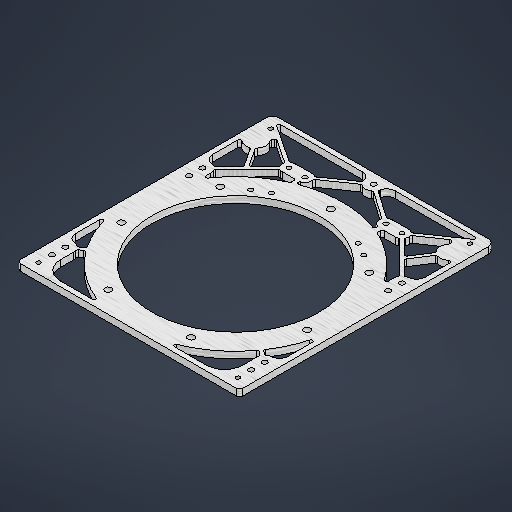
# Autodesk Inventor part: PLATE,SHOOTER,BOTTOM
Saved by Autodesk Inventor 2026.1 (Build 301233020, 233B)
## iProperties
Created: 2026-01-27
Part Number: PLATE,SHOOTER,BOTTOM
Material: Aluminum 7075
Document SubType Name: Sheet Metal
Designer: Owen L
Density: 2.81 g/cm^3
Appearance: Satin - Brushed Heavy
Mass: 376.468 g
Surface Area: 643.616 cm^2
Volume: 133.974 cm^3
Sheet Metal Rule: Default
Author: Owen L
Autodesk Inventor part; units mm, degrees
ref_plane "YZ Plane" through (0, 0, 0) normal (1, 0, 0) x (0, 1, 0)
ref_plane "XZ Plane" through (0, 0, 0) normal (0, 1, 0) x (-1, 0, 0)
ref_plane "XY Plane" through (0, 0, 0) normal (0, 0, 1) x (1, 0, 0)
sketch "Sketch1" plane through (0, 0, 0) normal (0, 1, 0) x (-1, 0, 0)
  line L0 (-105.7173, 139.7) -> (105.7173, 139.7)
  line L1 (105.7173, 139.7) -> (105.7173, -139.7)
  line L2 (105.7173, -139.7) -> (-105.7173, -139.7)
  line L3 (-105.7173, -139.7) -> (-105.7173, 139.7)
  line L4 (-105.7173, 139.7) -> (105.7173, -139.7) construction
  line L5 (105.7173, 139.7) -> (-105.7173, -139.7) construction
  circle A0 centre (0, 37.7949) radius 79.375
  point P0 (0, 0)
  dimension "d0" = 211.4347
  dimension "d1" = 279.4
  dimension "d2" = 158.75
  dimension "d3" = 101.9051
  measures "d0" distance of L1.end L2.end
  measures "d1" distance of L0.end L1.end
  measures "d2" diameter of A0
  measures "d3" distance from line of L0 A0.centre
extrude "Plate1" add sketch "Sketch1" along normal blind 6.35
sketch "Sketch2" plane through (0, 0, 0) normal (0, -1, 0) x (1, 0, 0)
  point P0 (0, 0)
  point P1 (-41.275, -37.3842)
  point P2 (-38.4175, -66.5942)
  point P3 (-53.6575, -66.5942)
  point P4 (-53.6575, -30.3992)
  dimension "d7" = 37.3842
  dimension "d11" = 41.275
  dimension "d12" = 6.985
  dimension "d13" = 29.21
  dimension "d14" = 2.8575
  dimension "d15" = 12.3825
  constraints: 1 horizontal alignment, 1 vertical alignment
  measures "d7" vertical distance of point (-41.275, -37.384) point (0, 0)
  measures "d11" horizontal distance of point (0, 0) point (-41.275, -37.384)
  measures "d12" vertical distance of point (-53.658, -30.399) point (-41.275, -37.384)
  measures "d13" vertical distance of point (-38.418, -66.594) point (-41.275, -37.384)
  measures "d14" horizontal distance of point (-38.418, -66.594) point (-41.275, -37.384)
  measures "d15" horizontal distance of point (-53.658, -66.594) point (-41.275, -37.384)
hole "Hole1" at (-41.275, 0, -37.3842) at (-38.4175, 0, -66.5942) at (-53.6575, 0, -66.5942) at (-53.6575, 0, -30.3992) direction (0, 1, 0) diameter 4.2926 depth 6.35 clearance for "Flat Head Machine Screw" size "M4" standard "Ansi Metric M Profile"
mirror "Mirror1" about plane through (0, 0, 0) normal (1, 0, 0) of "Hole1"
sketch "Sketch3" plane through (0, 6.35, 0) normal (0, 1, 0) x (1, 0, 0)
  line L0 (105.7173, -139.7) -> (-105.7173, -139.7) construction
  line L1 (105.7173, 139.7) -> (105.7173, -139.7) construction
  line L2 (-105.7173, 139.7) -> (105.7173, 139.7) construction
  line L3 (0, -139.7) -> (0, 139.7) construction
  point P0 (0, 0)
  point P1 (94.6048, -117.475)
  point P2 (94.6048, -104.775)
  point P3 (94.6048, 12.7)
  point P4 (94.6048, 25.4)
  point P5 (-87.3125, 139.7)
  point P6 (-94.6048, -117.475)
  point P7 (-94.6048, -104.775)
  point P8 (-94.6048, 12.7)
  point P9 (-94.6048, 25.4)
  dimension "d23" = 22.225
  dimension "d24" = 12.7
  dimension "d25" = 11.1125
  dimension "d26" = 12.7
  dimension "d60" = 152.4
  constraints: 4 symmetric about line, 3 vertical alignment, 2 end point, 2 midpoint
  measures "d23" distance from line of L0 point (94.605, -117.475)
  measures "d24" distance of point (94.605, -104.775) point (94.605, -117.475)
  measures "d25" distance from line of L1 point (94.605, -117.475)
  measures "d26" distance of point (94.605, 25.4) point (94.605, 12.7)
  measures "d60" distance from line of L0 point (94.605, 12.7)
hole "Hole2" at (94.6048, 6.35, 117.475) at (94.6048, 6.35, 104.775) at (94.6048, 6.35, -12.7) at (94.6048, 6.35, -25.4) at (-94.6048, 6.35, -25.4) at (-94.6048, 6.35, -12.7) at (-94.6048, 6.35, 104.775) at (-94.6048, 6.35, 117.475) direction (0, -1, 0) diameter 4.9784 depth 6.35 clearance for "Flat Head Machine Screw (82)" size "#10" standard "Ansi Unified Screw Threads"
sketch "Sketch5" plane through (0, 6.35, 0) normal (0, 1, 0) x (1, 0, 0)
  line L0 (-105.7173, 139.7) -> (-105.7173, -139.7) projected
  line L1 (105.7173, 139.7) -> (105.7173, -139.7) projected
  line L2 (-105.7173, 139.7) -> (105.7173, 139.7)
  line L3 (105.7173, 139.7) -> (105.7173, 102.9208)
  line L4 (105.7173, 102.9208) -> (-105.7173, 102.9208)
  line L5 (-105.7173, 102.9208) -> (-105.7173, 139.7)
  point P0 (0, 0)
  dimension "d61" = 36.7792
  constraints: 8 end point, 2 parallel, 1 horizontal, 1 perpendicular, 1 point on line
  measures "d61" distance of L2.end L3.end
extrude "Cut2" cut sketch "Sketch5" against normal blind 6.35
fillet "Corner Round3" radius 6.35 2 edges at (-105.7173, 3.175, -102.9208) (105.7173, 3.175, -102.9208)
fillet "Corner Round3" radius 3.175 2 edges at (-105.7173, 3.175, 139.7) (105.7173, 3.175, 139.7)
sketch "Sketch6" plane through (0, 6.35, 0) normal (0, 1, 0) x (1, 0, 0)
  line L0 (99.3673, 102.9208) -> (-99.3673, 102.9208) projected
  point P0 (0, 0)
  point P1 (0, 93.3958)
  dimension "d66" = 9.525
  constraints: 1 vertical alignment
  measures "d66" distance from line of L0 point (0, 93.396)
hole "Hole3" at (0, 6.35, -93.3958) direction (0, -1, 0) diameter 4.9784 end through all clearance for "Flat Head Machine Screw (82)" size "#10" standard "Ansi Unified Screw Threads"
sketch "Sketch7" plane through (0, 6.35, 0) normal (0, 1, 0) x (1, 0, 0)
  circle A0 centre (0, 93.3958) radius 2.4892 projected
  arc A1 (102.5423, -139.7) -> (105.7173, -136.525) centre (102.5423, -136.525) ccw projected
  line L0 (105.7173, 96.5708) -> (105.7173, -136.525) projected
  arc A2 (105.7173, 96.5708) -> (99.3673, 102.9208) centre (99.3673, 96.5708) ccw projected
  line L1 (99.3673, 102.9208) -> (-99.3673, 102.9208) projected
  arc A3 (-99.3673, 102.9208) -> (-105.7173, 96.5708) centre (-99.3673, 96.5708) ccw projected
  line L2 (-105.7173, -136.525) -> (-105.7173, 96.5708) projected
  arc A4 (-105.7173, -136.525) -> (-102.5423, -139.7) centre (-102.5423, -136.525) ccw projected
  line L3 (102.5423, -139.7) -> (-102.5423, -139.7) projected
  circle A5 centre (-94.6048, -117.475) radius 2.4892 projected
  circle A6 centre (-94.6048, -104.775) radius 2.4892 projected
  circle A7 centre (-94.6048, 12.7) radius 2.4892 projected
  circle A8 centre (-94.6048, 25.4) radius 2.4892 projected
  circle A9 centre (94.6048, 25.4) radius 2.4892 projected
  circle A10 centre (94.6048, 12.7) radius 2.4892 projected
  circle A11 centre (94.6048, -104.775) radius 2.4892 projected
  circle A12 centre (94.6048, -117.475) radius 2.4892 projected
  circle A13 centre (53.6575, 30.3992) radius 2.1463 projected
  circle A14 centre (53.6575, 66.5942) radius 2.1463 projected
  circle A15 centre (38.4175, 66.5942) radius 2.1463 projected
  circle A16 centre (41.275, 37.3842) radius 2.1463 projected
  circle A17 centre (-53.6575, 30.3992) radius 2.1463 projected
  circle A18 centre (-53.6575, 66.5942) radius 2.1463 projected
  circle A19 centre (-38.4175, 66.5942) radius 2.1463 projected
  circle A20 centre (-41.275, 37.3842) radius 2.1463 projected
  circle A21 centre (0, -37.7949) radius 79.375 projected
  arc A22 (-99.3673, 98.1583) -> (-100.9548, 96.5708) centre (-99.3673, 96.5708) ccw
  line L4 (-99.3673, 98.1583) -> (99.3673, 98.1583)
  arc A23 (100.9548, 96.5708) -> (99.3673, 98.1583) centre (99.3673, 96.5708) ccw
  line L5 (100.9548, 96.5708) -> (100.9548, -134.9375)
  line L6 (100.9548, -134.9375) -> (-100.9548, -134.9375)
  line L7 (-100.9548, -134.9375) -> (-100.9548, 96.5708)
  circle A24 centre (0, -37.7949) radius 101.6
  circle A25 centre (94.6048, 12.7) radius 7.9375
  circle A26 centre (94.6048, 25.4) radius 7.9375
  circle A27 centre (-94.6048, 12.7) radius 7.9375
  circle A28 centre (-94.6048, 25.4) radius 7.9375
  circle A29 centre (-94.6048, -117.475) radius 7.9375
  circle A30 centre (-94.6048, -104.775) radius 7.9375
  circle A31 centre (94.6048, -117.475) radius 7.9375
  circle A32 centre (94.6048, -104.775) radius 7.9375
  circle A33 centre (53.6575, 66.5942) radius 6.35
  circle A34 centre (38.4175, 66.5942) radius 6.35
  circle A35 centre (0, 93.3958) radius 7.9375
  circle A36 centre (-38.4175, 66.5942) radius 6.35
  circle A37 centre (-53.6575, 66.5942) radius 2.1463 projected
  circle A38 centre (-53.6575, 66.5942) radius 6.35
  line L8 (86.6673, -117.475) -> (86.6673, -104.775)
  line L9 (-86.6673, -117.475) -> (-86.6673, -104.775)
  line L10 (86.6673, 25.4) -> (86.6673, 12.7)
  line L11 (53.6575, 60.2442) -> (38.4175, 60.2442)
  line L12 (38.4175, 72.9442) -> (53.6575, 72.9442)
  line L13 (-38.4175, 72.9442) -> (-53.6575, 72.9442)
  line L14 (-53.6575, 60.2442) -> (-38.4175, 60.2442)
  line L15 (-86.6673, 12.7) -> (-86.6673, 25.4)
  arc A39 (-86.6673, -117.475) -> (-69.2048, -134.9375) centre (-69.2048, -117.475) ccw
  arc A40 (69.2048, -134.9375) -> (86.6673, -117.475) centre (69.2048, -117.475) ccw
  arc A41 (93.8111, 33.2977) -> (86.6673, 25.4) centre (94.6048, 25.4) ccw
  arc A42 (93.8111, 33.2977) -> (100.9548, 41.1954) centre (93.0173, 41.1954) ccw
  arc A43 (-86.6673, 25.4) -> (-93.8111, 33.2977) centre (-94.6048, 25.4) ccw
  arc A44 (-100.9548, 41.1954) -> (-93.8111, 33.2977) centre (-93.0173, 41.1954) ccw
  line L16 (0, 85.4583) -> (-7.6538, 85.4583) construction
  line L17 (0, 85.4583) -> (6.7881, 85.4583) construction
  arc A45 (-7.7771, 91.8083) -> (0, 85.4583) centre (0, 93.3958) ccw
  arc A46 (-7.7771, 91.8083) -> (-15.5543, 98.1583) centre (-15.5543, 90.2208) ccw
  arc A47 (0, 85.4583) -> (7.7771, 91.8083) centre (0, 93.3958) ccw
  arc A48 (15.5543, 98.1583) -> (7.7771, 91.8083) centre (15.5543, 90.2208) ccw
  arc A49 (-86.6673, -104.775) -> (-93.8111, -96.8773) centre (-94.6048, -104.775) ccw
  arc A50 (-100.9548, -88.9796) -> (-93.8111, -96.8773) centre (-93.0173, -88.9796) ccw
  arc A51 (93.8111, -96.8773) -> (86.6673, -104.775) centre (94.6048, -104.775) ccw
  arc A52 (93.8111, -96.8773) -> (100.9548, -88.9796) centre (93.0173, -88.9796) ccw
  arc A53 (1.4242, 91.3543) -> (-1.4242, 95.4373) centre (0, 93.3958) ccw
  line L18 (-53.6575, 66.5942) -> (-94.6048, 25.4) construction
  line L19 (-54.7834, 67.7134) -> (-95.7307, 26.5192)
  line L20 (-93.4789, 24.2808) -> (-52.5316, 65.475)
  arc A54 (-52.5316, 65.475) -> (-54.7834, 67.7134) centre (-53.6575, 66.5942) ccw
  arc A55 (-95.7307, 26.5192) -> (-93.4789, 24.2808) centre (-94.6048, 25.4) ccw
  line L21 (-53.6575, 66.5942) -> (-104.477, 100.341) construction
  line L22 (-52.7793, 67.9167) -> (-103.5988, 101.6634)
  line L23 (-105.3552, 99.0185) -> (-54.5357, 65.2717)
  arc A56 (-54.5357, 65.2717) -> (-52.7793, 67.9167) centre (-53.6575, 66.5942) ccw
  arc A57 (-103.5988, 101.6634) -> (-105.3552, 99.0185) centre (-104.477, 100.341) ccw
  line L24 (-38.4175, 66.5942) -> (-41.275, 37.3842) construction
  line L25 (-39.9975, 66.7488) -> (-42.855, 37.5388)
  line L26 (-39.695, 37.2296) -> (-36.8375, 66.4396)
  arc A58 (-36.8375, 66.4396) -> (-39.9975, 66.7488) centre (-38.4175, 66.5942) ccw
  arc A59 (-42.855, 37.5388) -> (-39.695, 37.2296) centre (-41.275, 37.3842) ccw
  line L27 (38.4175, 66.5942) -> (41.275, 37.3842) construction
  line L28 (36.2814, 66.3852) -> (39.1389, 37.1752)
  line L29 (43.4111, 37.5932) -> (40.5536, 66.8032)
  arc A60 (40.5536, 66.8032) -> (36.2814, 66.3852) centre (38.4175, 66.5942) ccw
  arc A61 (39.1389, 37.1752) -> (43.4111, 37.5932) centre (41.275, 37.3842) ccw
  line L30 (38.4175, 66.5942) -> (0, 93.3958) construction
  line L31 (39.3258, 67.8962) -> (0.9083, 94.6978)
  line L32 (-0.9083, 92.0938) -> (37.5092, 65.2922)
  arc A62 (37.5092, 65.2922) -> (39.3258, 67.8962) centre (38.4175, 66.5942) ccw
  arc A63 (0.9083, 94.6978) -> (-0.9083, 92.0938) centre (0, 93.3958) ccw
  line L33 (53.6575, 66.5942) -> (94.6048, 25.4) construction
  line L34 (52.5316, 65.475) -> (93.4789, 24.2808)
  line L35 (95.7307, 26.5192) -> (54.7834, 67.7134)
  arc A64 (54.7834, 67.7134) -> (52.5316, 65.475) centre (53.6575, 66.5942) ccw
  arc A65 (93.4789, 24.2808) -> (95.7307, 26.5192) centre (94.6048, 25.4) ccw
  line L36 (53.6575, 66.5942) -> (103.8575, 101.0609) construction
  line L37 (54.5561, 65.2855) -> (104.756, 99.7522)
  line L38 (102.9589, 102.3697) -> (52.7589, 67.9029)
  arc A66 (52.7589, 67.9029) -> (54.5561, 65.2855) centre (53.6575, 66.5942) ccw
  arc A67 (104.756, 99.7522) -> (102.9589, 102.3697) centre (103.8575, 101.0609) ccw
  line L39 (-38.4175, 66.5942) -> (0, 93.3958) construction
  line L40 (-37.5092, 65.2922) -> (0.9083, 92.0938)
  line L41 (-0.9083, 94.6978) -> (-39.3258, 67.8962)
  arc A68 (-39.3258, 67.8962) -> (-37.5092, 65.2922) centre (-38.4175, 66.5942) ccw
  arc A69 (0.9083, 92.0938) -> (-0.9083, 94.6978) centre (0, 93.3958) ccw
  line L42 (-94.6048, -104.775) -> (0, -37.7949) construction
  line L43 (-93.6875, -106.0706) -> (0.9173, -39.0906)
  line L44 (-0.9173, -36.4993) -> (-95.5222, -103.4794)
  arc A70 (-95.5222, -103.4794) -> (-93.6875, -106.0706) centre (-94.6048, -104.775) ccw
  arc A71 (0.9173, -39.0906) -> (-0.9173, -36.4993) centre (0, -37.7949) ccw
  line L45 (94.6048, -104.775) -> (0, -37.7949) construction
  line L46 (95.5222, -103.4794) -> (0.9173, -36.4993)
  line L47 (-0.9173, -39.0906) -> (93.6875, -106.0706)
  arc A72 (93.6875, -106.0706) -> (95.5222, -103.4794) centre (94.6048, -104.775) ccw
  arc A73 (0.9173, -36.4993) -> (-0.9173, -39.0906) centre (0, -37.7949) ccw
  circle A74 centre (-92.2553, 73.7108) radius 9.525
  line L48 (-92.2553, 73.7108) -> (-83.7232, 86.5594) construction
  line L49 (-90.9329, 72.8326) -> (-82.4007, 85.6812)
  line L50 (-85.0457, 87.4376) -> (-93.5778, 74.589)
  arc A75 (-93.5778, 74.589) -> (-90.9329, 72.8326) centre (-92.2553, 73.7108) ccw
  arc A76 (-82.4007, 85.6812) -> (-85.0457, 87.4376) centre (-83.7232, 86.5594) ccw
  line L51 (-92.2553, 73.7108) -> (-74.1312, 45.9971) construction
  line L52 (-93.5839, 72.8419) -> (-75.4598, 45.1282)
  line L53 (-72.8026, 46.866) -> (-90.9267, 74.5797)
  arc A77 (-90.9267, 74.5797) -> (-93.5839, 72.8419) centre (-92.2553, 73.7108) ccw
  arc A78 (-75.4598, 45.1282) -> (-72.8026, 46.866) centre (-74.1312, 45.9971) ccw
  line L54 (0, 102.9208) -> (0, -139.7) construction
  circle A79 centre (92.2553, 73.7108) radius 9.525
  line L55 (90.9329, 72.8326) -> (82.4007, 85.6812)
  line L56 (85.0457, 87.4376) -> (93.5778, 74.589)
  line L57 (92.2553, 73.7108) -> (74.1312, 45.9971) construction
  line L58 (93.5839, 72.8419) -> (75.4598, 45.1282)
  line L59 (72.8026, 46.866) -> (90.9267, 74.5797)
  point P0 (0, 0)
  point P1 (-74.1312, 45.9971)
  point P2 (-79.0672, 83.4676)
  point P3 (-100.4899, 97.6933)
  point P4 (-39.8463, 51.9892)
  point P5 (39.8463, 51.9892)
  point P6 (19.2088, 79.995)
  point P7 (74.1312, 45.9971)
  point P8 (78.7575, 83.8276)
  point P9 (-19.2088, 79.995)
  point P10 (-47.3024, -71.285)
  point P11 (47.3024, -71.285)
  point P12 (83.8284, -95.2002)
  point P13 (89.1748, -98.9855)
  point P14 (100.9548, -49.2265)
  point P15 (87.3402, -101.5767)
  point P16 (81.9938, -97.7915)
  point P17 (29.7638, -134.9375)
  point P18 (100.8696, 97.0839)
  point P19 (59.6247, 68.7656)
  point P20 (59.1179, 63.3528)
  point P21 (90.248, 32.0349)
  point P22 (93.8111, 33.2977)
  point P23 (87.9962, 29.7966)
  point P24 (56.8661, 61.1145)
  point P25 (41.1952, 60.2442)
  point P26 (41.7237, 54.8425)
  point P27 (86.6673, 15.2271)
  point P28 (57.8276, 71.383)
  point P29 (96.8252, 98.1583)
  point P30 (7.7771, 91.8083)
  point P31 (7.2866, 90.248)
  point P32 (34.2833, 71.414)
  point P33 (-5.47, 87.644)
  point P34 (-32.4667, 68.8101)
  point P35 (-37.4362, 60.3205)
  point P36 (-37.8091, 56.5079)
  point P37 (37.2249, 56.74)
  point P38 (36.8633, 60.4374)
  point P39 (32.4667, 68.8101)
  point P40 (5.47, 87.644)
  point P41 (-34.2833, 71.414)
  point P42 (-7.2866, 90.248)
  point P43 (-7.7771, 91.8083)
  point P44 (-98.3204, 98.1583)
  point P45 (-57.9012, 71.3179)
  point P46 (-59.6576, 68.6729)
  point P47 (-100.9548, 96.0965)
  point P48 (-93.8111, 33.2977)
  point P49 (-90.248, 32.0349)
  point P50 (-59.1179, 63.3528)
  point P51 (-41.1366, 55.1047)
  point P52 (-40.6338, 60.2442)
  point P53 (-56.8661, 61.1145)
  point P54 (-87.9962, 29.7966)
  point P55 (-86.6673, 15.2271)
  point P56 (-89.1748, -98.9855)
  point P57 (-83.8284, -95.2002)
  point P58 (-100.9548, -49.2265)
  point P59 (-29.7638, -134.9375)
  point P60 (-81.9938, -97.7915)
  point P61 (-87.3402, -101.5767)
  point P62 (-87.9893, 80.1351)
  point P63 (-83.1933, 59.854)
  point P64 (-76.1635, 46.2043)
  point P65 (-88.4436, 64.9818)
  point P66 (-100.9548, 69.8321)
  point P67 (-88.3824, 82.4129)
  point P68 (-85.9239, 86.1151)
  point P69 (-85.7864, 66.7195)
  point P70 (-73.8753, 48.5063)
  point P71 (-83.2789, 84.3587)
  point P72 (-85.7374, 80.6565)
  point P73 (85.7864, 66.7195)
  point P74 (85.7374, 80.6565)
  point P75 (82.9836, 84.8035)
  point P76 (73.8753, 48.5063)
  point P77 (100.9548, 69.8321)
  point P78 (88.4436, 64.9818)
  point P79 (76.1635, 46.2043)
  point P80 (85.6013, 86.6008)
  point P81 (88.3824, 82.4129)
  point P82 (-82.845, 87.8819)
  point P83 (-100.9548, 77.5895)
  point P84 (100.9548, 77.5895)
  dimension "d75" = 15.875
  dimension "d74" = 4.7625
  dimension "d76" = 12.7
  dimension "d77" = 7.9375
  dimension "d78" = 4.9784
  dimension "d79" = 3.175
  dimension "d80" = 3.175
  dimension "d81" = 3.175
  dimension "d82" = 4.2926
  dimension "d83" = 3.175
  dimension "d84" = 3.175
  dimension "d85" = 3.175
  dimension "d86" = 3.175
  dimension "d87" = 3.175
  dimension "d88" = 3.175
  dimension "d92" = 13.462
  dimension "d93" = 29.21
  dimension "d94" = 3.175
  dimension "d95" = 3.175
  dimension "d96" = 19.05
  dimension "d97" = 19.05
  dimension "d103" = 203.2
  constraints: 138 end point, 93 point on circle, 67 tangent, 48 centre point, 23 equal radius, 16 point on line, 15 midpoint, 14 coincident, 12 parallel, 10 symmetric about line, 5 vertical, 4 horizontal, 4 horizontal alignment, 1 perpendicular, 28 other
  measures "d74" distance between parallel lines of L2 L7
  measures "d76" diameter of A33
  measures "d77" radius of A42
  measures "d78" diameter of A53
  measures "d79" diameter of A55
  measures "d80" diameter of A57
  measures "d81" diameter of A59
  measures "d82" diameter of A61
  measures "d83" diameter of A63
  measures "d84" diameter of A65
  measures "d85" diameter of A67
  measures "d86" diameter of A69
  measures "d87" diameter of A71
  measures "d88" diameter of A73
  measures "d92" distance from line of L2 L48.start
  measures "d93" distance from line of L1 L48.start
  measures "d94" diameter of A76
  measures "d95" diameter of A78
  measures "d96" diameter of A74
  measures "d97" diameter of A79
  measures "d103" diameter of A24
extrude "Cut3" cut sketch "Sketch7" against normal blind 6.35 contours L32 A34 L28 A24 L26 A36 L40 A35 | A35 A48 L4 L38 A33 L12 A34 L31 | L41 A36 L13 A38 L22 L4 A46 A35 | L11 A33 L34 A26 L10 A24 L29 | A24 L15 A28 L20 A38 L14 L25 | L37 L55 A79 L59 L35 A33 | A38 L19 L53 A74 L49 L23 | L35 L58 A79 L5 A42 A26 | L5 A52 A32 L46 A24 | A28 A44 L7 A74 L52 L19 | A24 L44 A30 A50 L7 | L47 A32 L8 A40 L6 A24 | A24 L6 A39 L9 A30 L43
fillet "Corner Round4" radius 1.5875 58 edges at (-100.9548, 3.175, 49.2265) (-89.1748, 3.175, 98.9855) (-83.8284, 3.175, 95.2002) (-81.9938, 3.175, 97.7915) (-87.3402, 3.175, 101.5767) (-29.7638, 3.175, 134.9375) (87.3402, 3.175, 101.5767) (89.1748, 3.175, 98.9855) (81.9938, 3.175, 97.7915) (29.7638, 3.175, 134.9375) (83.8284, 3.175, 95.2002) (100.9548, 3.175, 49.2265) (87.9962, 3.175, -29.7966) (90.248, 3.175, -32.0349) (56.8661, 3.175, -61.1145) (59.1179, 3.175, -63.3528) (32.4667, 3.175, -68.8101) (36.8633, 3.175, -60.4374) (37.2249, 3.175, -56.74) (41.7237, 3.175, -54.8425) (-87.9962, 3.175, -29.7966) (-32.4667, 3.175, -68.8101) (-5.47, 3.175, -87.644) (5.47, 3.175, -87.644) (-41.1366, 3.175, -55.1047) (-86.6673, 3.175, -15.2271) (7.2866, 3.175, -90.248) (34.2833, 3.175, -71.414) (41.1952, 3.175, -60.2442) (57.8276, 3.175, -71.383) (-98.3204, 3.175, -98.1583) (-34.2833, 3.175, -71.414) (-7.2866, 3.175, -90.248) (59.6247, 3.175, -68.7656) (96.8252, 3.175, -98.1583) (86.6673, 3.175, -15.2271) (-59.6576, 3.175, -68.6729) (-57.9012, 3.175, -71.3179) (-37.4362, 3.175, -60.3205) (-37.8091, 3.175, -56.5079) (-40.6338, 3.175, -60.2442) (-59.1179, 3.175, -63.3528) (-90.248, 3.175, -32.0349) (-56.8661, 3.175, -61.1145) (-100.9548, 3.175, -69.8321) (-88.4436, 3.175, -64.9818) (-76.1635, 3.175, -46.2043) (-85.7864, 3.175, -66.7195) (-85.7374, 3.175, -80.6565) (-83.2789, 3.175, -84.3587) (-73.8753, 3.175, -48.5063) (85.7374, 3.175, -80.6565) (85.7864, 3.175, -66.7195) (73.8753, 3.175, -48.5063) (82.9836, 3.175, -84.8035) (76.1635, 3.175, -46.2043) (88.4436, 3.175, -64.9818) (100.9548, 3.175, -69.8321)
sketch "Sketch8" plane through (0, 0, 0) normal (0, -1, 0) x (1, 0, 0)
  circle A0 centre (0, 37.7949) radius 79.375 projected
  point P0 (0, 0)
  point P1 (0, -52.6926)
  point P2 (70.746, -18.6231)
  point P3 (88.2188, 57.9303)
  point P4 (39.2611, 119.3214)
  point P5 (-39.2611, 119.3214)
  point P6 (-88.2188, 57.9303)
  point P7 (-70.746, -18.6231)
  dimension "d100" = 360
  dimension "d102" = 90.4875
  constraints: 1 vertical alignment, 8 other
  measures "d102" distance of A0.centre point (0, -52.693)
hole "Hole4" at (0, 0, -52.6926) at (70.746, 0, -18.6231) at (88.2188, 0, 57.9303) at (39.2611, 0, 119.3214) at (-39.2611, 0, 119.3214) at (-88.2188, 0, 57.9303) at (-70.746, 0, -18.6231) direction (0, 1, 0) diameter 6.35 end through all
sketch "Sketch13" plane through (0, 6.35, 0) normal (0, 1, 0) x (1, 0, 0)
  circle A0 centre (-94.6048, -117.475) radius 2.4892 projected
  circle A1 centre (94.6048, -117.475) radius 2.4892 projected
  line L0 (102.5423, -139.7) -> (-102.5423, -139.7) projected
  line L1 (99.3673, 102.9208) -> (-99.3673, 102.9208) projected
  point P0 (0, 0)
  point P1 (-94.6048, -130.175)
  point P2 (94.6048, -130.175)
  point P3 (-94.6048, 90.2208)
  point P4 (94.6048, 90.2208)
  dimension "d135" = 9.525
  dimension "d136" = 12.7
  constraints: 4 vertical alignment, 2 horizontal alignment
  measures "d135" distance from line of L0 point (-94.605, -130.175)
  measures "d136" distance from line of L1 point (-94.605, 90.221)
hole "Hole6" at (-94.6048, 6.35, 130.175) at (94.6048, 6.35, 130.175) at (-94.6048, 6.35, -90.2208) at (94.6048, 6.35, -90.2208) direction (0, -1, 0) diameter 3.9624 depth 13.6144 tip angle 118 thread size "10-32 UNF" class "2B" standard "ANSI Unified Screw Threads"
equation "\"d21\" = Thickness"
equation "\"d34\" = Thickness"
equation "\"d4\" = Thickness"
equation "\"BendRadius\" = Thickness"
equation "\"BendReliefWidth\" = Thickness"
equation "\"BendReliefDepth\" = 0.5 * Thickness"
equation "\"CornerReliefSize\" = 4 * Thickness"
equation "\"MinimumRemnant\" = 2 * Thickness"
equation "\"TransitionRadius\" = BendRadius"
equation "\"JacobiRadiusSize\" = BendRadius"
equation "\"GapSize\" = Thickness"
equation "\"Thickness\" = 6.35"
body "Solid1"
